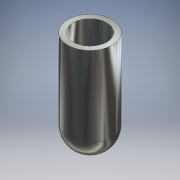
# Autodesk Inventor part: Toggle_Cap
Saved by Autodesk Inventor 2016 (Build 200138000, 138)
## iProperties
Created: 2016-04-13
Part Number: Toggle_Cap
Material: Nickel-Copper Alloy 400
Document SubType Name: Modeling
Designer: agmle
Density: 8.83 g/cm^3
Appearance: Chrome - Polished
Author: agmle
Autodesk Inventor part; units mm, degrees
ref_plane "YZ Plane" through (0, 0, 0) normal (1, 0, 0) x (0, 1, 0)
ref_plane "XZ Plane" through (0, 0, 0) normal (0, 1, 0) x (-1, 0, 0)
ref_plane "XY Plane" through (0, 0, 0) normal (0, 0, 1) x (1, 0, 0)
sketch "Sketch1" plane through (0, 0, 0) normal (0, 1, 0) x (-1, 0, 0)
  line L0 (0, 16) -> (0, 0) construction
  line L1 (2.69, 16) -> (3.55, 16)
  line L2 (3.55, 16) -> (3.55, 3.2833)
  arc A0 (1.35, 0) -> (3.55, 3.2833) centre (0, 3.2833) ccw
  line L3 (2.69, 16) -> (2.69, 3.2833)
  arc A1 (1.35, 0.9566) -> (2.69, 3.2833) centre (0, 3.2833) ccw
  line L4 (2.69, 16) -> (0, 16) construction
  line L5 (0, 0) -> (3.1469, 0) construction
  line L6 (1.35, 0) -> (1.35, 0.9566)
  dimension "d0" = 16
  dimension "d2" = 3.55
  dimension "d3" = 2.69
  dimension "d5" = 1.35
  constraints: 14 end point, 4 point on circle, 3 perpendicular, 3 vertical, 2 centre point, 2 coincident, 2 point on line, 2 tangent, 1 horizontal
  measures "d0" distance of L0.start L0.end
  measures "d2" distance between parallel lines of L0 L2
  measures "d3" distance between parallel lines of L0 L3
  measures "d5" distance between parallel lines of L0 L6
revolve "Revolution1" add sketch "Sketch1" angle 360 about axis through (0, 0, 16) along (0, 0, -1)
body "Solid1"
